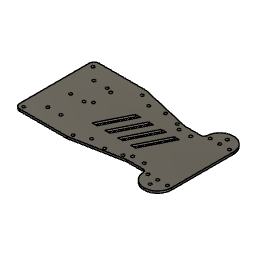
Car Frame v4 v6 (Autodesk Fusion 360 design; units mm, degrees)
Autodesk Fusion 360 part; units mm, degrees
sketch "Sketch1" plane through (0, 0, 0) normal (0, 0, 1) x (1, 0, 0)
  line L0 (0, 40) -> (155.0105, 40)
  line L1 (155.0105, 40) -> (155.0105, 81)
  line L2 (155.0105, 40) -> (155.0105, -1)
  circle A0 centre (155.0105, 72.125) radius 1.5
  circle A1 centre (165.0105, 72.1247) radius 1.5
  circle A2 centre (145.0105, 72.1252) radius 1.5
  circle A3 centre (155.0105, 79.925) radius 1.5
  circle A4 centre (145.0105, 7.8748) radius 1.5
  circle A5 centre (155.0105, 0.075) radius 1.5
  circle A6 centre (165.0105, 7.8753) radius 1.5
  line L3 (169.2354, 72.125) -> (169.2354, 40)
  arc A7 (140.8039, 7.1524) -> (169.2354, 7.875) centre (155.0105, 7.875) ccw
  line L4 (169.2354, 7.875) -> (169.2354, 40)
  circle A8 centre (155.0105, 7.875) radius 1.5
  line L5 (137.8078, 70) -> (120.9452, 70)
  line L6 (137.8078, 10) -> (120.9452, 10)
  line L7 (15, 5) -> (15, 77)
  line L8 (20, 82) -> (69, 82)
  line L9 (20, 0) -> (69, 0)
  line L10 (69, 82) -> (120.9452, 70)
  line L11 (69, 0) -> (120.9452, 10)
  circle A9 centre (20.1, 75.85) radius 1.5
  circle A10 centre (71.1, 75.85) radius 1.5
  circle A11 centre (20.1, 4.15) radius 1.5
  circle A12 centre (71.1, 4.15) radius 1.5
  circle A13 centre (32.95, 40) radius 1.5
  circle A14 centre (32.95, 63.85) radius 1.5
  circle A15 centre (32.95, 16.15) radius 1.5
  circle A16 centre (46.65, 63.85) radius 1.5
  circle A17 centre (46.65, 40) radius 1.5
  circle A18 centre (46.65, 16.15) radius 1.5
  circle A19 centre (52.2, 62) radius 1.5
  circle A20 centre (52.4253, 44.0014) radius 1.5
  circle A21 centre (133.0105, 64.05) radius 1.5
  circle A22 centre (121.0105, 64.05) radius 1.5
  circle A23 centre (121.0105, 15.95) radius 1.5
  circle A24 centre (133.0105, 15.95) radius 1.5
  circle A25 centre (84, 69.5) radius 1.5
  circle A26 centre (84, 10.5) radius 1.5
  arc A27 (169.2354, 72.125) -> (140.8039, 72.8476) centre (155.0105, 72.125) ccw
  circle A28 centre (99.5, 71.45) radius 1.5
  circle A29 centre (99.5, 8.55) radius 1.5
  circle A30 centre (115.0105, 68.05) radius 1.5
  circle A31 centre (115.0105, 11.95) radius 1.5
  line L12 (70, 25) -> (85, 55)
  line L13 (85, 55) -> (90, 55)
  line L14 (90, 55) -> (75, 25)
  line L15 (75, 25) -> (70, 25)
  line L16 (98.3333, 55) -> (103.3333, 55)
  line L17 (103.3333, 55) -> (88.3333, 25)
  line L18 (88.3333, 25) -> (83.3333, 25)
  line L19 (83.3333, 25) -> (98.3333, 55)
  line L20 (111.6667, 55) -> (116.6667, 55)
  line L21 (116.6667, 55) -> (101.6667, 25)
  line L22 (101.6667, 25) -> (96.6667, 25)
  line L23 (96.6667, 25) -> (111.6667, 55)
  line L24 (125, 55) -> (130, 55)
  line L25 (130, 55) -> (115, 25)
  line L26 (115, 25) -> (110, 25)
  line L27 (110, 25) -> (125, 55)
  arc A32 (20, 82) -> (15, 77) centre (20, 77) ccw
  arc A33 (15, 5) -> (20, 0) centre (20, 5) ccw
  arc A34 (140.8039, 7.1524) -> (137.8078, 10) centre (137.8078, 7) ccw
  arc A35 (137.8078, 70) -> (140.8039, 72.8476) centre (137.8078, 73) ccw
  point P0 (155.0105, 7.875)
  point P1 (140.9452, 70)
  point P2 (15, 0)
  point P3 (15, 82)
  dimension "d6" = 41
  dimension "d7" = 3
  dimension "d8" = 32.125
  dimension "d9" = 3
  dimension "d10" = 10
  dimension "d11" = 3
  dimension "d12" = 10
  dimension "d13" = 3
  dimension "d14" = 7.8
  dimension "d18" = 20
  dimension "d20" = 54
  dimension "d21" = 54
  dimension "d22" = 3
  dimension "d23" = 3
  dimension "d24" = 6.15
  dimension "d25" = 6.15
  dimension "d26" = 5.1
  dimension "d27" = 51
  dimension "d30" = 3
  dimension "d31" = 17.95
  dimension "d32" = 3
  dimension "d33" = 17.95
  dimension "d34" = 23.85
  dimension "d37" = 13.7
  dimension "d38" = 0
  dimension "d39" = 3
  dimension "d40" = 20
  dimension "d41" = 37.2
  dimension "d42" = 3
  dimension "d43" = 18
  dimension "d44" = 24.05
  dimension "d45" = 3
  dimension "d48" = -12
  dimension "d49" = 0
  dimension "d51" = 10
  dimension "d52" = 22
  dimension "d53" = 3
  dimension "d54" = 69
  dimension "d55" = 12.5
  dimension "d56" = 82
  dimension "d57" = 60
  dimension "d58" = 3
  dimension "d59" = 15.5
  dimension "d60" = 31.45
  dimension "d61" = 3
  dimension "d62" = 4
  dimension "d63" = 6
  dimension "d66" = 40
  dimension "d67" = 0
  dimension "d68" = 5
  dimension "d69" = 5
  dimension "d70" = 3
  dimension "d71" = 3
  dimension "d76" = 71.7
  dimension "d77" = 71.7
  constraint perpendicular L0 L1
  constraint symmetric L1.start L0 L2.start
  constraint symmetric L0 L1.end L2.end
  constraint coincident L1 A0.centre
  constraint coincident L1 A3.centre
  constraint symmetric L0 A0.centre P0
  constraint symmetric L0 A1 A6
  constraint symmetric L0 A2 A4
  constraint symmetric L0 A3 A5
  constraint vertical L3
  constraint symmetric L0 L3.start A7.end
  constraint symmetric L0 L3.end L4.end
  constraint symmetric L0 A0 A8
  constraint horizontal L5
  constraint symmetric L0 L5.end L6.end
  constraint perpendicular L7 L8
  constraint perpendicular L7 L9
  constraint symmetric L0 A9 A11
  constraint symmetric L0 A10 A12
  constraint coincident L0 A13.centre
  constraint symmetric L0 A14 A15
  constraint symmetric L0 A21 A24
  constraint symmetric L0 A22 A23
  constraint symmetric L0 A25 A26
  constraint concentric A0 A27
  constraint symmetric L0 A28 A29
  constraint symmetric L0 A30 A31
  constraint parallel L0 L13
  constraint parallel L12 L14
  constraint parallel L0 L15
  constraint coincident P3 L7
  constraint coincident P3 L8
  constraint tangent L7 A32
  constraint tangent L8 A32
  constraint coincident P2 L7
  constraint coincident P2 L9
  constraint tangent L7 A33
  constraint tangent L9 A33
  constraint tangent L6 A34
  constraint tangent A7 A34
  constraint coincident P1 L5
  constraint coincident P1 A27
  constraint tangent L5 A35
  constraint tangent A27 A35
  measures "d6" distance of L0.end L1.end
  measures "d7" diameter of A0
  measures "d8" distance of L0.end A0.centre
  measures "d9" diameter of A1
  measures "d10" distance of A0.centre A1.centre
  measures "d11" diameter of A2
  measures "d12" distance of A0.centre A2.centre
  measures "d13" diameter of A3
  measures "d14" distance of A0.centre A3.centre
  measures "d18" distance of P1 L5.end
  measures "d20" distance of P3 L8.end
  measures "d21" distance of P2 L9.end
  measures "d22" diameter of A9
  measures "d23" diameter of A10
  measures "d24" distance of L8 A9.centre
  measures "d25" distance of L8 A10.centre
  measures "d26" distance of L7 A9.centre
  measures "d27" distance of A9.centre A10.centre
  measures "d30" diameter of A13
  measures "d31" distance of L7 A13.centre
  measures "d32" diameter of A14
  measures "d33" distance of L7 A14.centre
  measures "d34" distance of L0 A14.centre
  measures "d39" diameter of A19
  measures "d40" distance of L8 A19.centre
  measures "d41" distance of L7 A19.centre
  measures "d42" diameter of A20
  measures "d43" distance of A19.centre A20.centre
  measures "d44" distance of L0 A21.centre
  measures "d45" diameter of A21
  measures "d51" distance of A0.centre A2.centre
  measures "d52" distance of L1 A21.centre
  measures "d53" diameter of A25
  measures "d54" distance of L7 A25.centre
  measures "d55" distance of L8 A25.centre
  measures "d56" distance of P2 P3
  measures "d58" diameter of A28
  measures "d59" horizontal distance of A25.centre A28.centre
  measures "d60" distance of L0 A28.centre
  measures "d61" diameter of A30
  measures "d62" vertical distance of A22.centre A30.centre
  measures "d63" horizontal distance of A22.centre A30.centre
  measures "d68" radius of A32
  measures "d69" radius of A33
  measures "d70" radius of A34
  measures "d71" radius of A35
  measures "d76" distance of A9.centre A11.centre
  measures "d77" distance of A10.centre A12.centre
extrude "Extrude1" add sketch "Sketch1" along normal blind 2
move_body "Move1" bodies 1 to x (1, 0, 0) y (0, 1, 0) z (0, 0, 1) at (-64.9596, -41.0567, 43.5725)
